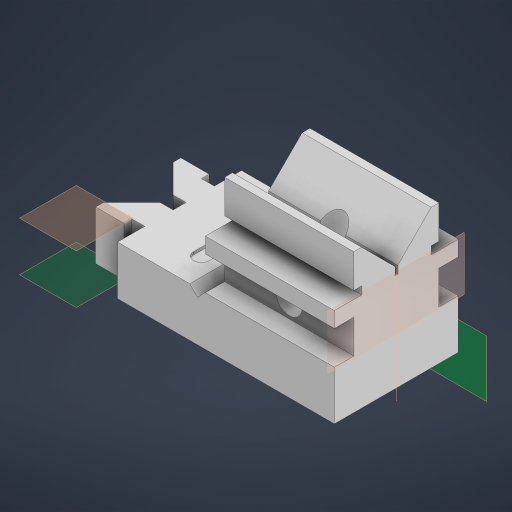
# Autodesk Inventor part: Część30
Saved by Autodesk Inventor 2023 (Build 270158000, 158)
## iProperties
Created: 2023-05-09
Part Number: Część30
Material: Ogólny
Document SubType Name: Modeling
Designer: Adam
Density: 1 g/cm^3
Appearance: Domyślna
Author: Adam
Autodesk Inventor part; units mm, degrees
ref_plane "YZ Plane" through (0, 0, 0) normal (1, 0, 0) x (0, 1, 0)
ref_plane "XZ Plane" through (0, 0, 0) normal (0, 1, 0) x (-1, 0, 0)
ref_plane "XY Plane" through (0, 0, 0) normal (0, 0, 1) x (1, 0, 0)
sketch "Szkic1" plane through (0, 0, 0) normal (0, 1, 0) x (-1, 0, 0)
  line L0 (-100, 0) -> (-100, -48)
  line L1 (-11, -7.5) -> (0, -7.5)
  line L2 (-11, -40.5) -> (0, -40.5)
  line L3 (-16, 0) -> (-16, -10.5)
  line L4 (-16, -10.5) -> (-11, -10.5)
  line L5 (-16, -48) -> (-16, -37.5)
  line L6 (-16, -37.5) -> (-11, -37.5)
  line L7 (-11, -21.5) -> (-16, -21.5)
  line L8 (-16, -21.5) -> (-16, -26.5)
  line L9 (-16, -26.5) -> (-11, -26.5)
  line L10 (0, -7.5) -> (0, -14.4549)
  line L11 (0, -40.5) -> (0, -37.5)
  line L12 (0, -7.5) -> (0, -10.5)
  line L13 (0, -10.5) -> (-11, -21.5)
  line L14 (-11, -26.5) -> (0, -37.5)
  line L15 (-100, 0) -> (-100, -48)
  line L16 (-100, 0) -> (-16, 0)
  line L17 (-16, -10.5) -> (-16, 0)
  line L18 (-16, -10.5) -> (-11, -10.5)
  line L19 (-11, -10.5) -> (-11, -7.5)
  line L20 (-11, -7.5) -> (0, -7.5)
  line L21 (0, -7.5) -> (0, -10.5)
  line L22 (0, -10.5) -> (-11, -21.5)
  line L23 (-11, -21.5) -> (-16, -21.5)
  line L24 (-16, -21.5) -> (-16, -26.5)
  line L25 (-16, -26.5) -> (-11, -26.5)
  line L26 (-11, -26.5) -> (0, -37.5)
  line L27 (0, -37.5) -> (0, -40.5)
  line L28 (0, -40.5) -> (-11, -40.5)
  line L29 (-11, -40.5) -> (-11, -37.5)
  line L30 (-11, -37.5) -> (-16, -37.5)
  line L31 (-16, -37.5) -> (-16, -48)
  line L32 (-16, -48) -> (-100, -48)
  line L33 (-100, -48) -> (-100, 0)
  point P0 (0, 0)
  dimension "d1" = 48
  dimension "d2" = 11
  dimension "d5" = 5
  dimension "d6" = 10.5
  dimension "d7" = 10.5
  dimension "d8" = 5
  dimension "d10" = 11
  dimension "d11" = 5
  dimension "d12" = 5
  dimension "d15" = 3
  dimension "d16" = 3
  dimension "d77" = 90
  constraints: 68 end point, 12 collinear, 5 perpendicular, 2 point on line, 1 horizontal, 1 vertical
  measures "d1" distance of L0.end L0.start
  measures "d2" distance of L1.end L1.start
  measures "d5" distance of L4.end L3.end
  measures "d6" distance of L3.end L3.start
  measures "d7" distance of L5.start L5.end
  measures "d8" distance of L7.end L8.end
  measures "d10" distance between parallel lines of L7 L4
  measures "d11" distance of L8.end L9.end
  measures "d12" distance of L7.start L7.end
  measures "d15" distance of L12.end L1.end
  measures "d16" distance from line of L11.end L2
  measures "d77" angle of L14 L13
ref_plane "Płaszczyzna konstrukcyjna6" through (0, 19, 0) normal (0, 1, 0) x (1, 0, 0)
ref_plane "Płaszczyzna konstrukcyjna2" through (100, 0, -48) normal (0, 0, -1) x (-1, 0, 0)
ref_plane "Płaszczyzna konstrukcyjna3" through (100, 0, -48) normal (0, 0, -1) x (-1, 0, 0)
ref_plane "Płaszczyzna konstrukcyjna1" through (100, 0, 0) normal (1, 0, 0) x (0, 0, -1)
sketch "Szkic6" plane through (100, 0, 0) normal (1, 0, 0) x (0, 0, -1)
  line L0 (0, 19) -> (48, 19) projected
  line L1 (7.5, 19) -> (40.5, 19)
  line L2 (7.5, 19) -> (7.5, 32)
  line L3 (7.5, 32) -> (0, 32)
  line L4 (0, 32) -> (0, 38)
  line L5 (0, 38) -> (10.5, 38)
  line L6 (10.5, 38) -> (10.5, 41)
  line L7 (10.5, 41) -> (7.5, 41)
  line L8 (0, 0) -> (48, 0) projected
  line L9 (40.5, 19) -> (40.5, 32)
  line L10 (40.5, 32) -> (48, 32)
  line L11 (48, 32) -> (48, 38)
  line L12 (48, 38) -> (37.5, 38)
  line L13 (37.5, 38) -> (37.5, 41)
  line L14 (37.5, 41) -> (40.5, 41)
  line L15 (24.0424, 40.4576) -> (10.5, 54)
  line L16 (23.97, 39) -> (43.1219, 39) construction
  line L17 (24.0424, 40.4576) -> (37.5, 53.9152)
  line L18 (7.5, 41) -> (7.5, 52.5)
  line L19 (7.5, 54) -> (10.5, 54)
  line L20 (37.5, 53.9152) -> (40.5, 53.9152)
  line L21 (40.5, 52.4987) -> (40.5, 41)
  line L22 (23.5, 38) -> (24.5, 38)
  line L23 (23.5, 38) -> (23.5, 41)
  line L24 (24.5, 38) -> (24.5, 41)
  line L25 (7.5, 52.5) -> (7.5, 54)
  line L26 (40.5, 52.4987) -> (40.5, 53.9152)
  point P0 (10.5, 39.5)
  point P1 (24.5, 40.9152)
  point P2 (39, 53.9152)
  dimension "d27" = 33
  dimension "d28" = 7.5
  dimension "d30" = 10.5
  dimension "d32" = 38
  dimension "d33" = 6
  dimension "d36" = 10.5
  dimension "d49" = 3
  dimension "d50" = 3
  dimension "d51" = 135
  dimension "d52" = 1
  dimension "d54" = 3
  dimension "d55" = 13
  dimension "d56" = 3
  dimension "d57" = 3
  dimension "d74" = 53.9152
  dimension "d75" = 13
  constraints: 52 end point, 14 perpendicular, 5 point on line, 5 vertical, 2 horizontal, 2 midpoint, 1 collinear, 1 equal length
  measures "d27" distance of L1.start L1.end
  measures "d28" distance of L0.start L1.start
  measures "d30" distance of L4.end L5.end
  measures "d32" distance between parallel lines of L8 L5
  measures "d33" distance between parallel lines of L5 L3
  measures "d36" distance of L11.end L12.end
  measures "d49" distance of L6.end L7.end
  measures "d50" distance of L13.end L14.end
  measures "d51" angle of L16 L15
  measures "d52" distance of L22.start L22.end
  measures "d54" distance of L22.start L23.end
  measures "d55" distance between parallel lines of L13 L24
  measures "d56" distance of L19.start L15.end
  measures "d57" distance of L17.end L20.end
  measures "d74" distance from line of L8 point (39, 53.915)
  measures "d75" distance of L1.end L9.end
extrude "Wyciągnięcie proste4" add sketch "Szkic6" against normal blind 50 contours L2 L3 L4 L5 L6 L7 L18 L25 L19 L15 L23 L22 L24 L17 L20 L26 L21 L14 L13 L12 L11 L10 L9 L0
ref_plane "Płaszczyzna konstrukcyjna4" through (0, 0, 0) normal (0, -1, 0) x (1, 0, 0)
sketch "Szkic8" plane through (0, 0, 0) normal (0, -1, 0) x (1, 0, 0)
  line L0 (100, -23.5) -> (50, -23.5) projected
  point P0 (0, 0)
  point P1 (75, -23.5)
  constraints: 1 midpoint
hole "Otwór1" at (75, 0, -23.5) direction (0, 1, 0) diameter 10 end through all
sketch "Szkic9" plane through (100, 19, -40.5) normal (0, 0, -1) x (-1, 0, 0)
  line L0 (0, -19) -> (100, -19) projected
  point P0 (25, 6)
  point P1 (84, -19)
  dimension "d76" = 25
  measures "d76" distance from line of L0 point (25, 6)
hole "Otwór2" at (75, 25, -40.5) direction (0, 0, 1) diameter 10 end through all
extrude "Wyciągnięcie proste5" add sketch "Szkic1" along normal blind 19
sketch "Szkic10" plane through (0, 19, 0) normal (0, 1, 0) x (1, 0, 0)
  line L0 (37, 36.5) -> (37, 11.5) construction
  line L1 (40, 36.5) -> (40, 11.5)
  line L2 (34, 11.5) -> (34, 36.5)
  arc A0 (40, 36.5) -> (34, 36.5) centre (37, 36.5) ccw
  arc A1 (34, 11.5) -> (40, 11.5) centre (37, 11.5) ccw
  line L3 (100, 57.6) -> (100, -9.6) projected
  line L4 (16, 0) -> (100, 0) projected
  point P0 (0, 0)
  point P1 (37, 24)
  dimension "d80" = 25
  dimension "d82" = 63
  dimension "d83" = 3
  dimension "d84" = 11.5
  constraints: 8 end point, 4 point on circle, 4 tangent, 2 centre point, 1 midpoint, 1 parallel, 1 vertical
  measures "d80" distance of L0.start L0.end
  measures "d82" distance from line of L3 point (37, 24)
  measures "d83" radius of A0
  measures "d84" distance from line of L4 L0.end
extrude "Wyciągnięcie proste6" cut sketch "Szkic10" against normal blind 1
sketch "Szkic11" plane through (16, 0, 0) normal (0, 0, 1) x (1, 0, 0)
  line L0 (34, 19) -> (31, 16)
  line L1 (31, 16) -> (28, 19)
  line L2 (28, 19) -> (34, 19)
  line L3 (84, 19) -> (0, 19) projected
  point P0 (-16, 0)
  dimension "d89" = 3
  constraints: 6 end point, 1 collinear, 1 perpendicular
  measures "d89" horizontal distance of L0.end L1.end
extrude "Wyciągnięcie proste7" cut sketch "Szkic11" against normal through all
